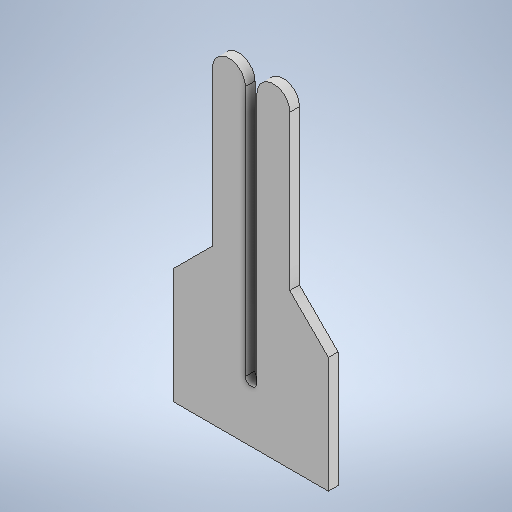
# Autodesk Inventor part: clip
Saved by Autodesk Inventor 2025.2 (Build 292293000, 293)
## iProperties
Created: 2025-02-17
Part Number: clip
Material: Generic
Document SubType Name: Modeling
Designer: kenne
Density: 1 g/cm^3
Appearance: Default
Author: kenne
Autodesk Inventor part; units mm, degrees
ref_plane "YZ Plane" through (0, 0, 0) normal (1, 0, 0) x (0, 1, 0)
ref_plane "XZ Plane" through (0, 0, 0) normal (0, 1, 0) x (-1, 0, 0)
ref_plane "XY Plane" through (0, 0, 0) normal (0, 0, 1) x (1, 0, 0)
sketch "Sketch1" plane through (0, 0, 0) normal (0, 0, 1) x (1, 0, 0)
  line L0 (40, 0) -> (40, -60)
  line L1 (40, -60) -> (-40, -60)
  line L2 (-40, -60) -> (-40, 0)
  line L3 (40, 0) -> (40, 20) construction
  line L4 (-40, 0) -> (-20, 0) construction
  line L5 (-20, 100) -> (-20, 20)
  line L6 (-20, 20) -> (-40, 0)
  line L7 (-3, 100) -> (-3, -30)
  line L8 (-3, 100) -> (3, 100) construction
  line L9 (3, 100) -> (3, -30)
  line L10 (20, 100) -> (20, 20)
  line L11 (20, 20) -> (40, 0)
  arc A0 (-3, 100) -> (-20, 100) centre (-11.5, 100) ccw
  arc A1 (20, 100) -> (3, 100) centre (11.5, 100) ccw
  arc A2 (-3, -30) -> (3, -30) centre (0, -30) ccw
  point P0 (0, 0)
  dimension "d2" = 60
  dimension "d3" = 80
  dimension "d4" = 20
  dimension "d5" = 20
  dimension "d9" = 6
  dimension "d10" = 17
  dimension "d11" = 8.5
  dimension "d12" = 8.5
  constraints: 24 end point, 6 point on circle, 6 vertical, 3 centre point, 3 horizontal, 2 tangent
  measures "d2" distance of L0.start L0.end
  measures "d3" distance of L0.end L1.end
  measures "d4" distance of L0.start L3.end
  measures "d5" distance of L2.end L4.end
  measures "d9" distance of L7.start L8.end
  measures "d10" distance of L8.end L10.start
  measures "d11" radius of A0
  measures "d12" radius of A1
extrude "Extrusion1" add sketch "Sketch1" along normal blind 5
body "Solid1"
